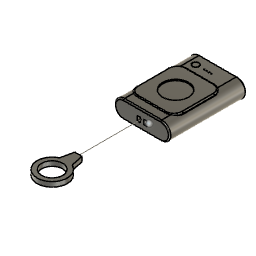
Watch battery bank_ (Autodesk Fusion 360 design; units mm, degrees)
Autodesk Fusion 360 part; units mm, degrees
sketch "Sketch1" plane through (0, 0, 0) normal (0, 0, 1) x (1, 0, 0)
  line L0 (0, 0) -> (-46, 0)
  line L1 (-46, 0) -> (-46, 64)
  line L2 (-46, 64) -> (0, 64)
  line L3 (0, 64) -> (0, 0)
  dimension "d1" = 46
  dimension "d2" = 64
  constraint horizontal L0
  constraint vertical L1
  constraint horizontal L2
  constraint vertical L3
  constraint coincident L0.start L3.end
  measures "d1" distance of L0.start L0.end
  measures "d2" distance of L0.start L2.end
extrude "Extrude1" add sketch "Sketch1" along normal blind 15 makes body 1
fillet "Fillet1" radius 7.5 4 edges at (0, 32, 15) (0, 32, 0) (-46, 32, 15) (-46, 32, 0) on bodies 1
sketch "Sketch2" plane through (0, 0, 0) normal (0, -1, 0) x (1, 0, 0)
  arc A0 (-38.5, 15) -> (-38.5, 0) centre (-38.5, 7.5) ccw
  line L0 (-38.5, 0) -> (-7.5, 0)
  arc A1 (-7.5, 0) -> (-7.5, 15) centre (-7.5, 7.5) ccw
  line L1 (-7.5, 15) -> (-38.5, 15)
  line L2 (-21.5, 8.9167) -> (-19, 8.9167)
  line L3 (-19, 8.9167) -> (-19, 4.9167)
  line L4 (-19, 4.9167) -> (-21.5, 4.9167)
  line L5 (-21.5, 4.9167) -> (-21.5, 8.9167)
  line L6 (-24.5, 8.9167) -> (-27, 8.9167)
  line L7 (-24.5, 4.9167) -> (-24.5, 8.9167)
  line L8 (-27, 4.9167) -> (-24.5, 4.9167)
  line L9 (-27, 8.9167) -> (-27, 4.9167)
  dimension "d7" = 2.5
  dimension "d8" = 4
  dimension "d9" = 11.5
  constraint horizontal L2
  constraint vertical L3
  constraint horizontal L4
  constraint vertical L5
  measures "d7" distance of L2.start L2.end
  measures "d8" distance of L2.start L4.end
  measures "d9" distance of A1.centre L3
extrude "Extrude2" cut sketch "Sketch2" against normal blind 5 contours L2 L3 L4 L5 | L6 L7 L8 L9 bodies 1
fillet "Fillet2" radius 1 8 edges at (-23, 64, 0) (0, 64, 7.5) (-23, 64, 15) (-46, 64, 7.5) (-23, 0, 0) (-46, 0, 7.5) (-23, 0, 15) (0, 0, 7.5) on bodies 1
sketch "Sketch3" plane through (0, 0, 15) normal (0, 0, 1) x (-1, 0, 0)
  line L0 (38.5, -1) -> (7.5, -1)
  line L1 (7.5, -1) -> (7.5, -63)
  line L2 (7.5, -63) -> (38.5, -63)
  line L3 (38.5, -63) -> (38.5, -1)
  line L4 (3.75, -7.5) -> (42.25, -7.5)
  line L5 (42.25, -7.5) -> (42.25, -48.5)
  line L6 (42.25, -48.5) -> (3.75, -48.5)
  line L7 (3.75, -48.5) -> (3.75, -7.5)
  dimension "d14" = 38.5
  dimension "d15" = 41
  dimension "d16" = 6.5
  dimension "d17" = 31
  dimension "d18" = 3.75
  constraint horizontal L4
  constraint vertical L5
  constraint horizontal L6
  constraint vertical L7
  measures "d14" distance of L4.start L4.end
  measures "d15" distance of L4.start L6.end
  measures "d16" distance of L0 L4
  measures "d17" distance of L0.start L0.end
  measures "d18" distance of L1 L4.start
extrude "Extrude3" add sketch "Sketch3" against normal blind 2 contours L3 L4 L5 L6 | L1 L3 L4 L6 | L1 L4 L6 L7 bodies 1
extrude "Extrude4" add sketch "Sketch3" along normal blind 0.5 contours L3 L4 L5 L6 | L1 L3 L4 L6 | L1 L4 L6 L7 bodies 1
fillet "Fillet3" radius 7.5 4 edges at (-42.25, 7.5, 14.7476) (-3.75, 7.5, 14.7476) (-3.75, 48.5, 14.7476) (-42.25, 48.5, 14.7476) on bodies 1
fillet "Fillet4" radius 1 8 edges at (-23, 48.5, 15.5) (-5.9467, 46.3033, 15.5) (-3.75, 28, 15.5) (-5.9467, 9.6967, 15.5) (-23, 7.5, 15.5) (-40.0533, 9.6967, 15.5) (-42.25, 28, 15.5) (-40.0533, 46.3033, 15.5) on bodies 1
sketch "Sketch4" plane through (0, 0, 15.5) normal (0, 0, 1) x (-1, 0, 0)
  arc A0 (40.3336, -44.3277) -> (41.25, -41) centre (34.75, -41) ccw
  line L0 (41.25, -41) -> (41.25, -15)
  arc A1 (41.25, -15) -> (40.3336, -11.6723) centre (34.75, -15) ccw
  spline S0 degree 3 poles (38.067, -9.2548) (38.6296, -9.5796) (39.1148, -10.0315) (39.8315, -10.8928) (40.0981, -11.2772) (40.3336, -11.6723) knots 2.811721 2.811721 2.811721 2.811721 3.006867 3.006867 3.144848 3.144848 3.144848 3.144848
  arc A2 (38.067, -9.2548) -> (34.75, -8.366) centre (34.75, -15) ccw
  line L1 (34.75, -8.366) -> (11.25, -8.366)
  arc A3 (11.25, -8.366) -> (7.933, -9.2548) centre (11.25, -15) ccw
  spline S1 degree 3 poles (5.6664, -11.6723) (5.7918, -11.4619) (5.926, -11.2551) (6.3611, -10.6403) (6.6878, -10.2501) (7.3244, -9.6603) (7.6177, -9.4369) (7.933, -9.2548) knots 1.037587 1.037587 1.037587 1.037587 1.110653 1.110653 1.261742 1.261742 1.370985 1.370985 1.370985 1.370985
  arc A4 (5.6664, -11.6723) -> (4.75, -15) centre (11.25, -15) ccw
  line L2 (4.75, -15) -> (4.75, -41)
  arc A5 (4.75, -41) -> (5.6664, -44.3277) centre (11.25, -41) ccw
  spline S2 degree 3 poles (7.933, -46.7452) (7.3512, -46.4093) (6.8543, -45.9395) (6.1449, -45.073) (5.8916, -44.7055) (5.6664, -44.3277) knots 2.84648 2.84648 2.84648 2.84648 3.047896 3.047896 3.179832 3.179832 3.179832 3.179832
  arc A6 (7.933, -46.7452) -> (11.25, -47.634) centre (11.25, -41) ccw
  line L3 (11.25, -47.634) -> (34.75, -47.634)
  arc A7 (34.75, -47.634) -> (38.067, -46.7452) centre (34.75, -41) ccw
  spline S3 degree 3 poles (40.3336, -44.3277) (40.2559, -44.458) (40.1754, -44.5862) (39.7858, -45.1742) (39.4378, -45.6144) (38.7464, -46.2846) (38.4206, -46.541) (38.067, -46.7452) knots 1.037165 1.037165 1.037165 1.037165 1.082397 1.082397 1.248779 1.248779 1.371275 1.371275 1.371275 1.371275
  circle A8 centre (23, -28) radius 10.75
  dimension "d27" = 21.5
  dimension "d29" = 39.2679
  dimension "d30" = 36.5
  dimension "d31" = 19.634
  dimension "d32" = 19.634
  dimension "d33" = 18.25
  measures "d27" diameter of A8
  measures "d29" distance of L1 L3
  measures "d30" distance of L0 L2
  measures "d31" distance of L1 A8.centre
  measures "d32" distance of L3 A8.centre
  measures "d33" distance of L0 A8.centre
extrude "Extrude5" cut sketch "Sketch4" against normal blind 1 contours A8 bodies 1
sketch "Sketch5" plane through (0, 0, 15) normal (0, 0, 1) x (-1, 0, 0)
  line L0 (34.75, -48.5) -> (11.25, -48.5)
  arc A0 (7.5, -47.4952) -> (11.25, -48.5) centre (11.25, -41) ccw
  line L1 (7.5, -47.4952) -> (7.5, -63)
  line L2 (7.5, -63) -> (38.5, -63)
  line L3 (38.5, -63) -> (38.5, -47.4952)
  arc A1 (34.75, -48.5) -> (38.5, -47.4952) centre (34.75, -41) ccw
  circle A2 centre (33.25, -55) radius 2.5
  circle A3 centre (26.25, -55) radius 0.5
  circle A4 centre (24.25, -55) radius 0.5
  circle A5 centre (22.25, -55) radius 0.5
  circle A6 centre (20.25, -55) radius 0.5
  circle A7 centre (33.25, -55) radius 2.75
  dimension "d36" = 5
  dimension "d37" = 6.5
  dimension "d38" = 1
  dimension "d39" = 7
  dimension "d40" = 1
  dimension "d41" = 2
  dimension "d42" = 1
  dimension "d43" = 1
  dimension "d44" = 2
  dimension "d45" = 2
  dimension "d46" = 6.5
  dimension "d47" = 6.5
  dimension "d48" = 6.5
  dimension "d49" = 6.5
  dimension "d50" = 5.5
  dimension "d51" = 5.25
  constraint concentric A2 A7
  measures "d36" diameter of A2
  measures "d37" distance of L0 A2.centre
  measures "d38" diameter of A3
  measures "d39" distance of A2.centre A3.centre
  measures "d40" diameter of A4
  measures "d41" horizontal distance of A3.centre A4.centre
  measures "d42" diameter of A5
  measures "d43" diameter of A6
  measures "d44" distance of A5.centre A6.centre
  measures "d45" horizontal distance of A4.centre A5.centre
  measures "d46" distance of L0 A3.centre
  measures "d47" distance of L0 A4.centre
  measures "d48" distance of L0 A5.centre
  measures "d49" distance of L0 A6.centre
  measures "d50" diameter of A7
  measures "d51" distance of L3 A2.centre
extrude "Extrude6" cut sketch "Sketch5" against normal blind 0.8 contours A3 | A4 | A5 | A6 | A7 bodies 1
sketch "Sketch6" plane through (0, 0, 0) normal (0, 0, 1) x (1, 0, 0)
  line L0 (-26.3317, -38.4902) -> (-20.3317, -38.4902)
  line L1 (-28.5817, -48.9902) -> (-18.0817, -48.9902)
  line L2 (-26.3317, -38.4902) -> (-28.5817, -48.9902)
  line L3 (-20.3317, -38.4902) -> (-18.0817, -48.9902)
  circle A0 centre (-23.3317, -60.3343) radius 12.5
  circle A1 centre (-23.3317, -60.3343) radius 8.75
  dimension "d54" = 6
  dimension "d55" = 10.5
  dimension "d56" = 10.5
  dimension "d57" = 10.7384
  dimension "d58" = 10.7384
  dimension "d59" = 25
  dimension "d60" = 12.5
  dimension "d61" = 12.5
  dimension "d62" = 17.5
  constraint horizontal L0
  constraint parallel L0 L1
  constraint concentric A0 A1
  measures "d54" distance of L0.start L0.end
  measures "d55" distance of L1.start L1.end
  measures "d56" distance of L0 L1
  measures "d57" distance of L0.start L1.start
  measures "d58" distance of L0.end L1.end
  measures "d59" diameter of A0
  measures "d60" distance of L1.end A0.centre
  measures "d61" distance of L1.start A0.centre
  measures "d62" diameter of A1
extrude "Extrude7" add sketch "Sketch6" along normal blind 4 separate body makes body 2
sketch "Sketch7" plane through (0, -38.4902, 0) normal (0, 1, 0) x (-1, 0, 0)
  line L0 (20.3317, 0) -> (26.3317, 0)
  line L1 (26.3317, 0) -> (26.3317, 4)
  line L2 (26.3317, 4) -> (20.3317, 4)
  line L3 (20.3317, 4) -> (20.3317, 0)
  circle A0 centre (22.3317, 2) radius 0.75
  circle A1 centre (24.3317, 2) radius 0.75
  dimension "d65" = 1.5
  dimension "d66" = 1.5
  dimension "d67" = 2
  dimension "d68" = 2
  dimension "d70" = 6
  dimension "d71" = 2
  dimension "d72" = 4
  dimension "d73" = 2
  measures "d65" diameter of A0
  measures "d66" diameter of A1
  measures "d67" distance of L3 A0.centre
  measures "d68" distance of A0.centre A1.centre
  measures "d70" distance of L1 L3
  measures "d71" distance of L2 A0.centre
  measures "d72" distance of L0.end L1.end
  measures "d73" distance of L0 A1.centre
extrude "Extrude8" cut sketch "Sketch7" against normal blind 2 contours A0 | A1 bodies 2
move_body "Move1" bodies 2 to x (1, 0, 0) y (0, 1, 0) z (0, 0, 1) at (0.3317, 38.4902, 5.5)
move_body "Move2" bodies 1 to x (1, 0, 0) y (0, 1, 0) z (0, 0, 1) at (0, 53, 0)
sketch "Sketch8" plane through (0, 0, 0) normal (0, 0, 1) x (1, 0, 0)
  line L0 (-26, 0) -> (-25.75, 0)
  line L1 (-25.75, 0) -> (-25.75, 53)
  line L2 (-25.75, 53) -> (-26, 53)
  line L3 (-26, 53) -> (-26, 0)
  dimension "d76" = 0.25
  dimension "d77" = 53
  constraint horizontal L0
  constraint vertical L1
  constraint horizontal L2
  constraint vertical L3
  measures "d76" distance of L0.start L0.end
  measures "d77" distance of L0.start L2.end
revolve "Revolve1" add sketch "Sketch8" angle 360 about axis through (-25.75, 0, 0) along (0, 1, 0) separate body makes body 3
move_body "Move3" bodies 3 to x (1, 0, 0) y (0, 1, 0) z (0, 0, 1) at (1.75, 0, 7.5)
sketch "Sketch10" plane through (0, 0, 0) normal (0, 0, 1) x (1, 0, 0)
  line L0 (-26, 61) -> (-25, 61)
  constraint horizontal L0
equation "d9 = 19 mm - 7.5 mm"
equation "d18 = ( d14 - d17 ) / 2"
equation "d31 = ( d29 ) / 2"
equation "d33 = d30 / 2"
equation "d37 = 4 mm + d36 / 2"
equation "d39 = 4 mm + d36 / 2 + d38 / 2"
equation "d44 = d41"
equation "d45 = d41"
equation "d46 = d37"
equation "d47 = d46"
equation "d48 = d37"
equation "d49 = d46"
equation "d51 = 2.5 mm + d50 / 2"
equation "d57 = d58"
equation "d67 = d70 / 3"
equation "d68 = d70 / 3"
equation "d71 = d72 / 2"
equation "d73 = d72 / 2"
